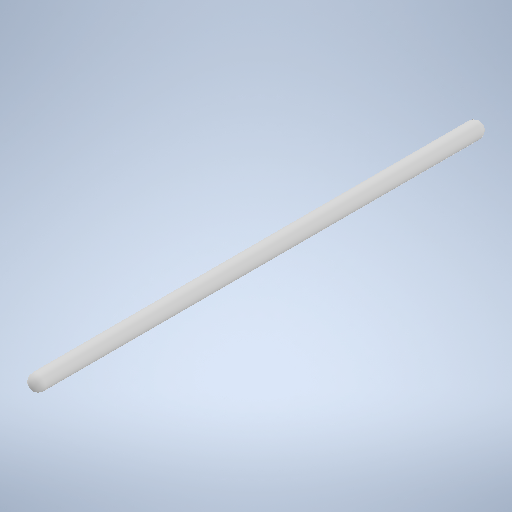
# Autodesk Inventor part: Stösselstange
Saved by Autodesk Inventor 2025 (Build 290162010, 162A)
## iProperties
Created: 2024-07-17
Part Number: Stösselstange
Material: Generic
Document SubType Name: Modeling
Designer: ffogue
Density: 1 g/cm^3
Appearance: Default
Author: ffogue
Autodesk Inventor part; units mm, degrees
ref_plane "YZ Plane" through (0, 0, 0) normal (1, 0, 0) x (0, 1, 0)
ref_plane "XZ Plane" through (0, 0, 0) normal (0, 1, 0) x (-1, 0, 0)
ref_plane "XY Plane" through (0, 0, 0) normal (0, 0, 1) x (1, 0, 0)
sketch "Sketch1" plane through (0, 0, 0) normal (0, 1, 0) x (-1, 0, 0)
  arc A0 (1, -1) -> (0, 0) centre (0, -1) ccw
  line L0 (1, -1) -> (1, -57)
  arc A1 (0, -58) -> (1, -57) centre (0, -57) ccw
  line L1 (0, 0) -> (0, -58)
  dimension "d0" = 58
  dimension "d1" = 2
  constraints: 4 end point, 4 point on circle, 2 centre point, 2 tangent, 2 vertical, 2 vertical alignment
  measures "d0" distance of L1.end L1.start
  measures "d1" diameter of L0 L1
revolve "Revolution1" add sketch "Sketch1" angle 360 about axis through (0, 0, 0) along (0, 0, -1)
body "Solid1"
